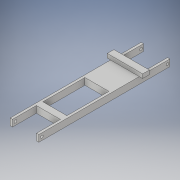
# Autodesk Inventor part: Mousetrap Car
Saved by Autodesk Inventor 2017 (Build 210142000, 142)
## iProperties
Created: 2017-09-07
Part Number: Mousetrap Car
Material: Generic
Document SubType Name: Modeling
Designer: 168416
Density: 1 g/cm^3
Appearance: Default
Author: 168416
Autodesk Inventor part; units mm, degrees
ref_plane "YZ Plane" through (0, 0, 0) normal (1, 0, 0) x (0, 1, 0)
ref_plane "XZ Plane" through (0, 0, 0) normal (0, 1, 0) x (-1, 0, 0)
ref_plane "XY Plane" through (0, 0, 0) normal (0, 0, 1) x (1, 0, 0)
sketch "Sketch1" plane through (0, 0, 0) normal (0, 1, 0) x (-1, 0, 0)
  line L0 (146.7721, -144.7877) -> (142.3271, -144.7877)
  line L1 (142.3271, -144.7877) -> (142.3271, 134.6123)
  line L2 (142.3271, 134.6123) -> (146.7721, 134.6123)
  line L3 (146.7721, 134.6123) -> (146.7721, -144.7877)
  line L4 (96.6071, -144.7877) -> (96.6071, 134.6123)
  line L5 (96.6071, 134.6123) -> (92.1621, 134.6123)
  line L6 (92.1621, 134.6123) -> (92.1621, -144.7877)
  line L7 (92.1621, -144.7877) -> (96.6071, -144.7877)
  line L8 (142.3271, -91.4477) -> (96.6071, -91.4477)
  line L9 (142.3271, -25.4077) -> (96.6071, -25.4077)
  point P0 (0, 0)
  dimension "d0" = 4.445
  dimension "d1" = 279.4
  dimension "d2" = 4.445
  dimension "d3" = 45.72
  dimension "d4" = 66.04
  dimension "d5" = 53.34
  constraints: 20 end point, 7 perpendicular, 4 point on line, 1 horizontal, 1 parallel, 1 vertical
  measures "d0" distance of L0.start L0.end
  measures "d1" distance of L0.end L1.end
  measures "d2" distance between parallel lines of L6 L4
  measures "d3" distance between parallel lines of L4 L1
  measures "d4" distance between parallel lines of L9 L8
  measures "d5" distance from line of L4.start L8
extrude "Extrusion1" add sketch "Sketch1" along normal blind 12.7
sketch "Sketch2" plane through (0, 12.7, 0) normal (0, 1, 0) x (1, 0, 0)
  line L0 (-142.3271, 91.4477) -> (-142.3271, 144.7877) projected
  line L1 (-142.3271, 91.4477) -> (-146.7721, 91.4477)
  line L2 (-146.7721, 144.7877) -> (-146.7721, -134.6123) projected
  line L3 (-153.1221, 91.4477) -> (-146.7721, 91.4477)
  line L4 (-96.6071, 91.4477) -> (-142.3271, 91.4477) projected
  line L5 (-96.6071, 91.4477) -> (-92.1621, 91.4477)
  line L6 (-92.1621, -134.6123) -> (-92.1621, 144.7877) projected
  line L7 (-92.1621, 91.4477) -> (-85.8121, 91.4477)
  line L8 (-85.8121, 91.4477) -> (-85.8121, 78.7477)
  line L9 (-85.8121, 78.7477) -> (-153.1221, 78.7477)
  line L10 (-153.1221, 78.7477) -> (-153.1221, 91.4477)
  point P0 (0, 0)
  dimension "d8" = 6.35
  dimension "d9" = 6.35
  dimension "d10" = 12.7
  constraints: 14 end point, 3 horizontal, 3 point on line, 2 perpendicular, 1 collinear, 1 parallel
  measures "d8" distance of L3.start L1.end
  measures "d9" distance of L5.end L7.end
  measures "d10" distance of L7.end L8.end
extrude "Extrusion2" add sketch "Sketch2" along normal blind 7.62
sketch "Sketch3" plane through (-146.7721, 0, -144.7877) normal (-1, 0, 0) x (0, 0, 1)
  line L0 (279.4, 0) -> (279.4, 12.7) projected
  circle A0 centre (251.46, 6.35) radius 2.54
  point P0 (144.7877, 0)
  dimension "d15" = 5.08
  constraints: 1 centre point
  measures "d15" diameter of A0
extrude "Extrusion3" cut sketch "Sketch3" against normal blind 25400
sketch "Sketch4" plane through (-146.7721, 0, -144.7877) normal (-1, 0, 0) x (0, 0, 1)
  line L0 (0, 0) -> (0, 12.7) projected
  circle A0 centre (12.7052, 6.35) radius 2.54
  point P0 (144.7877, 0)
  dimension "d19" = 5.08
  constraints: 1 centre point
  measures "d19" diameter of A0
extrude "Extrusion4" cut sketch "Sketch4" against normal blind 25400
sketch "Sketch5" plane through (0, 12.7, 0) normal (0, 1, 0) x (1, 0, 0)
  line L0 (-146.7721, 144.7877) -> (-146.7721, -134.6123) projected
  line L1 (-142.3271, -134.6123) -> (-142.3271, 25.4077) projected
  line L2 (-142.3271, -66.9401) -> (-96.6071, -66.9401)
  line L3 (-96.6071, 25.4077) -> (-96.6071, -134.6123) projected
  line L4 (-96.6071, -54.6023) -> (-142.3271, -54.6023)
  line L5 (-142.3271, -54.6023) -> (-142.3271, -66.9401)
  point P0 (0, 0)
  constraints: 6 end point, 2 horizontal, 2 point on line, 1 midpoint, 1 parallel
extrude "Extrusion5" add sketch "Sketch5" against normal blind 12.7
sketch "Sketch6" plane through (-146.7721, 0, 134.6123) normal (0, 0, 1) x (1, 0, 0)
  line L0 (0, 12.7) -> (4.445, 12.7) projected
  line L1 (4.445, 0) -> (4.445, 12.7) projected
  line L2 (0, 12.7) -> (4.445, 12.7)
  line L3 (4.445, 12.7) -> (4.445, 0)
  line L4 (4.445, 0) -> (0, 0)
  line L5 (0, 0) -> (0, 12.7)
  line L6 (50.165, 0) -> (50.165, 12.7) projected
  line L7 (54.61, 0) -> (54.61, 12.7) projected
  line L8 (50.165, 12.7) -> (54.61, 12.7)
  line L9 (54.61, 12.7) -> (54.61, 0)
  line L10 (54.61, 0) -> (50.165, 0)
  line L11 (50.165, 0) -> (50.165, 12.7)
  point P0 (146.7721, 0)
  constraints: 16 end point, 4 parallel, 2 horizontal, 2 perpendicular
extrude "Extrusion6" cut sketch "Sketch6" against normal blind 22.225
sketch "Sketch7" plane through (-92.1621, 0, -144.7877) normal (0, 0, -1) x (-1, 0, 0)
  line L0 (50.165, 0) -> (50.165, 12.7) projected
  line L1 (54.61, 12.7) -> (50.165, 12.7)
  line L2 (50.165, 12.7) -> (50.165, 0)
  line L3 (50.165, 0) -> (54.61, 0)
  line L4 (54.61, 0) -> (54.61, 12.7)
  line L5 (4.445, 0) -> (4.445, 12.7) projected
  line L6 (0, 0) -> (4.445, 0) projected
  line L7 (4.445, 12.7) -> (0, 12.7)
  line L8 (0, 12.7) -> (0, 0)
  line L9 (0, 0) -> (4.445, 0)
  line L10 (4.445, 0) -> (4.445, 12.7)
  point P0 (-92.1621, 0)
  constraints: 16 end point, 4 parallel, 2 horizontal, 2 perpendicular
extrude "Extrusion7" cut sketch "Sketch7" against normal blind 7.9375
body "Solid1"
